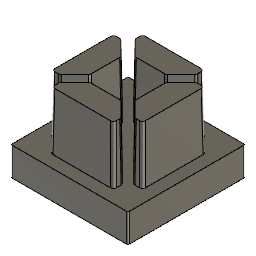
7) PLA Extrusion Caps (Autodesk Fusion 360 design; units mm, degrees)
Autodesk Fusion 360 part; units mm, degrees
ref_plane "WorkPlane1" through (0, 0, 0) normal (0, 0, 1) x (1, 0, 0)
sketch "Sketch1" plane through (0, 0, 0) normal (0, 0, 1) x (1, 0, 0)
  line L0 (10.25, 10.25) -> (-10.25, 10.25)
  line L1 (-10.25, 10.25) -> (-10.25, -10.25)
  line L2 (-10.25, -10.25) -> (10.25, -10.25)
  line L3 (10.25, -10.25) -> (10.25, 10.25)
  line L4 (10.25, 10.25) -> (-10.25, -10.25) construction
  line L5 (-10.25, 10.25) -> (10.25, -10.25) construction
  line L6 (3.75, 3.75) -> (-3.75, 3.75)
  line L7 (-3.75, 3.75) -> (-3.75, -3.75)
  line L8 (-3.75, -3.75) -> (3.75, -3.75)
  line L9 (3.75, -3.75) -> (3.75, 3.75)
  line L10 (3.75, 3.75) -> (-3.75, -3.75) construction
  line L11 (-3.75, 3.75) -> (3.75, -3.75) construction
  line L12 (8.1, 8.1) -> (-8.1, 8.1)
  line L13 (-8.1, 8.1) -> (-8.1, -8.1)
  line L14 (-8.1, -8.1) -> (8.1, -8.1)
  line L15 (8.1, -8.1) -> (8.1, 8.1)
  line L16 (8.1, 8.1) -> (-8.1, -8.1) construction
  line L17 (-8.1, 8.1) -> (8.1, -8.1) construction
  line L18 (10.25, 10.25) -> (5.55, 10.25)
  line L19 (5.55, 10.25) -> (5.55, 5.55)
  line L20 (5.55, 5.55) -> (10.25, 5.55)
  line L21 (10.25, 5.55) -> (10.25, 10.25)
  line L22 (2.7601, 3.75) -> (5.55, 6.5399)
  line L23 (3.75, 2.7601) -> (6.5399, 5.55)
  line L24 (4.155, 5.145) -> (5.145, 4.155)
  line L25 (-5.55, 5.55) -> (-5.55, 10.25)
  line L26 (-10.25, 5.55) -> (-5.55, 5.55)
  line L27 (-3.75, 2.7601) -> (-6.5399, 5.55)
  line L28 (-2.7601, 3.75) -> (-5.55, 6.5399)
  line L29 (-5.55, -5.55) -> (-10.25, -5.55)
  line L30 (-5.55, -10.25) -> (-5.55, -5.55)
  line L31 (-2.7601, -3.75) -> (-5.55, -6.5399)
  line L32 (-3.75, -2.7601) -> (-6.5399, -5.55)
  line L33 (5.55, -5.55) -> (5.55, -10.25)
  line L34 (10.25, -5.55) -> (5.55, -5.55)
  line L35 (3.75, -2.7601) -> (6.5399, -5.55)
  line L36 (2.7601, -3.75) -> (5.55, -6.5399)
  point P0 (4.65, 4.65)
  dimension "d2" = 20.5
  dimension "d3" = 20.5
  dimension "d4" = 7.5
  dimension "d5" = 7.5
  dimension "d6" = 16.2
  dimension "d7" = 16.2
  dimension "d8" = 4.7
  dimension "d9" = 4.7
  dimension "d10" = 1.4
  dimension "d12" = 360
  constraint horizontal L0
  constraint perpendicular L0 L1
  constraint parallel L0 L2
  constraint parallel L1 L3
  constraint coincident L4 origin
  constraint coincident L5 origin
  constraint horizontal L6
  constraint perpendicular L6 L7
  constraint parallel L6 L8
  constraint parallel L7 L9
  constraint coincident L10 origin
  constraint coincident L11 origin
  constraint horizontal L12
  constraint perpendicular L12 L13
  constraint parallel L12 L14
  constraint parallel L13 L15
  constraint coincident L16 origin
  constraint coincident L17 origin
  constraint horizontal L18
  constraint vertical L19
  constraint horizontal L20
  constraint vertical L21
  constraint coincident L6 L22.start
  constraint coincident L19 L22.end
  constraint parallel L4 L22
  constraint coincident L9 L23.start
  constraint coincident L20 L23.end
  constraint parallel L4 L23
  constraint midpoint L22 L24.start
  constraint midpoint L23 L24.end
  constraint midpoint L24 P0
  constraint coincident L4 P0
  measures "d2" distance of L1.end L2.end
  measures "d3" distance of L0.end L1.end
  measures "d4" distance of L7.end L8.end
  measures "d5" distance of L6.end L7.end
  measures "d6" distance of L13.end L14.end
  measures "d7" distance of L12.end L13.end
  measures "d8" distance of L0.start L18.end
  measures "d9" distance of L0.start L20.end
  measures "d10" distance of L22 L23
extrude "Extrude1" add sketch "Sketch1" against normal blind 5 makes body 1
extrude "Extrude2" add sketch "Sketch1" along normal blind 10 draft -1 separate body contours L6 L12 L19 L22 L25 L28 makes body 2
sketch "Sketch2" plane through (0, 0, -5) normal (0, 0, -1) x (1, 0, 0)
  line L0 (10.25, -10.25) -> (10.25, 10.25)
  line L1 (10.25, 10.25) -> (-10.25, 10.25)
  line L2 (-10.25, 10.25) -> (-10.25, -10.25)
  line L3 (-10.25, -10.25) -> (10.25, -10.25)
  circle A0 centre (0, 0) radius 2.1
  line L4 (2.0063, 3.475) -> (-2.0063, 3.475)
  line L5 (-2.0063, 3.475) -> (-4.0126, 0)
  line L6 (-4.0126, 0) -> (-2.0063, -3.475)
  line L7 (-2.0063, -3.475) -> (2.0063, -3.475)
  line L8 (2.0063, -3.475) -> (4.0126, 0)
  line L9 (4.0126, 0) -> (2.0063, 3.475)
  dimension "d17" = 4.2
  dimension "d18" = 3.475
  constraint coincident A0.centre origin
  constraint horizontal L4
  measures "d17" diameter of A0
  measures "d18" distance of A0.centre L9
fillet "Fillet1" radius 0.5 6 edges at (2.7239, 3.8373, 5) (-2.7239, 3.8373, 5) (-5.4627, 6.5761, 5) (5.4627, 6.5761, 5) (5.4627, 8.0127, 5) (-5.4627, 8.0127, 5) on bodies 2
pattern_circular "C-Pattern1" count 4 over 360 about axis through (0, 0, 1.75) along (0, 0, 1) of bodies 2 makes body 3 at (-8.0418, 1.6252, 3.3333) makes body 4 at (-1.6252, -8.0418, 3.3333) makes body 5 at (8.0418, -1.6252, 3.3333)
combine "Combine1" operation add target body 5 tool bodies 4 3 2 1
fillet "Fillet2" radius 0.2 4 edges at (10.25, -10.25, -2.5) (10.25, 10.25, -2.5) (-10.25, 10.25, -2.5) (-10.25, -10.25, -2.5) on bodies 5
equation "d18 = ( 6.95 / 2 ) * 1 mm"
named bodies: "Extrusion Cap"
